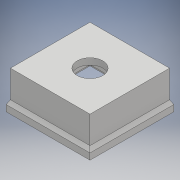
# Autodesk Inventor part: lupa_camera_mount
Saved by Autodesk Inventor 2018 (Build 220112000, 112)
## iProperties
Created: 2018-01-19
Part Number: lupa_camera_mount
Material: Generic
Document SubType Name: Modeling
Designer: matth
Density: 1 g/cm^3
Appearance: Default
Author: matth
Autodesk Inventor part; units mm, degrees
ref_plane "YZ Plane" through (0, 0, 0) normal (1, 0, 0) x (0, 1, 0)
ref_plane "XZ Plane" through (0, 0, 0) normal (0, 1, 0) x (-1, 0, 0)
ref_plane "XY Plane" through (0, 0, 0) normal (0, 0, 1) x (1, 0, 0)
sketch "Sketch1" plane through (0, 0, 0) normal (0, 0, 1) x (1, 0, 0)
  line L0 (-11.7234, 6.1825) -> (23.1766, 6.1825)
  line L1 (23.1766, 6.1825) -> (23.1766, -28.7175)
  line L2 (23.1766, -28.7175) -> (-11.7234, -28.7175)
  line L3 (-11.7234, -28.7175) -> (-11.7234, 6.1825)
  line L4 (-13.2234, 7.6825) -> (24.6766, 7.6825)
  line L5 (24.6766, 7.6825) -> (24.6766, -30.2175)
  line L6 (24.6766, -30.2175) -> (-13.2234, -30.2175)
  line L7 (-13.2234, -30.2175) -> (-13.2234, 7.6825)
  point P0 (0, 0)
  dimension "d0" = 34.9
  dimension "d1" = 34.9
  dimension "d2" = 37.9
  dimension "d3" = 37.9
  dimension "d4" = 1.5
  dimension "d5" = 1.5
  constraints: 16 end point, 4 parallel, 2 horizontal, 2 perpendicular
  measures "d0" distance of L1.end L2.end
  measures "d1" distance of L0.end L1.end
  measures "d2" distance of L5.end L6.end
  measures "d3" distance of L4.end L5.end
  measures "d4" distance between parallel lines of L4 L0
  measures "d5" distance between parallel lines of L7 L3
extrude "Extrusion1" add sketch "Sketch1" along normal blind 15
sketch "Sketch2" plane through (0, 0, 15) normal (0, 0, 1) x (1, 0, 0)
  line L0 (-13.2234, -30.2175) -> (-13.2234, 7.6825) projected
  line L1 (-13.2234, -30.2175) -> (24.6766, -30.2175) projected
  line L2 (-13.2234, 7.6825) -> (24.6766, 7.6825)
  line L3 (24.6766, 7.6825) -> (24.6766, -30.2175)
  line L4 (24.6766, -30.2175) -> (-13.2234, -30.2175)
  line L5 (-13.2234, -30.2175) -> (-13.2234, 7.6825)
  point P0 (0, 0)
  constraints: 8 end point, 2 parallel, 1 horizontal, 1 perpendicular
extrude "Extrusion2" add sketch "Sketch2" along normal blind 1
sketch "Sketch3" plane through (0, 0, 16) normal (0, 0, 1) x (1, 0, 0)
  circle A0 centre (5.7266, -11.2675) radius 6.1
  line L0 (-13.2234, 7.6825) -> (-13.2234, -30.2175) projected
  line L1 (-13.2234, -30.2175) -> (24.6766, -30.2175) projected
  point P0 (0, 0)
  dimension "d10" = 12.2
  dimension "d11" = 18.95
  dimension "d12" = 18.95
  dimension "d13" = 37.9
  constraints: 1 centre point
  measures "d10" diameter of A0
  measures "d11" distance from line of L0 A0.centre
  measures "d12" distance from line of L1 A0.centre
  measures "d13" distance of L0.start L0.end
extrude "Extrusion3" cut sketch "Sketch3" against normal blind 1
sketch "Sketch4" plane through (0, 0, 15) normal (0, 0, -1) x (-1, 0, 0)
  circle A0 centre (-5.7266, -11.2675) radius 6.1 projected
  circle A1 centre (-5.7266, -11.2675) radius 7.1
  point P0 (0, 0)
  dimension "d16" = 14.2
  constraints: 1 centre point, 1 coincident
  measures "d16" diameter of A1
extrude "Extrusion4" add sketch "Sketch4" along normal blind 2
sketch "Sketch5" plane through (0, 0, 0) normal (0, 0, -1) x (-1, 0, 0)
  line L0 (-24.6766, 7.6825) -> (-24.6766, -30.2175) projected
  line L1 (-24.6766, -30.2175) -> (13.2234, -30.2175) projected
  line L2 (13.2234, -30.2175) -> (13.2234, 7.6825) projected
  line L3 (13.2234, 7.6825) -> (-24.6766, 7.6825) projected
  line L4 (-25.6766, -31.2175) -> (14.2234, -31.2175)
  line L5 (14.2234, -31.2175) -> (14.2234, 8.6825)
  line L6 (14.2234, 8.6825) -> (-25.6766, 8.6825)
  line L7 (-25.6766, 8.6825) -> (-25.6766, -31.2175)
  point P0 (0, 0)
  dimension "d19" = 1
  dimension "d20" = 1
  dimension "d21" = 1
  dimension "d22" = 1
  constraints: 8 end point, 2 parallel, 1 horizontal, 1 perpendicular
  measures "d19" distance between parallel lines of L4 L1
  measures "d20" distance between parallel lines of L5 L2
  measures "d21" distance between parallel lines of L6 L3
  measures "d22" distance between parallel lines of L7 L0
extrude "Extrusion5" add sketch "Sketch5" along normal blind 2
sketch "Sketch6" plane through (0, 0, 0) normal (0, 0, 1) x (1, 0, 0)
  line L0 (-13.2234, 7.6825) -> (24.6766, 7.6825) projected
  line L1 (24.6766, 7.6825) -> (24.6766, -30.2175) projected
  line L2 (24.6766, -30.2175) -> (-13.2234, -30.2175) projected
  line L3 (-13.2234, -30.2175) -> (-13.2234, 7.6825) projected
  line L4 (25.6766, -31.2175) -> (-14.2234, -31.2175) projected
  line L5 (25.6766, 8.6825) -> (25.6766, -31.2175) projected
  line L6 (-14.2234, 8.6825) -> (25.6766, 8.6825) projected
  line L7 (-14.2234, -31.2175) -> (-14.2234, 8.6825) projected
  circle A0 centre (5.7266, -11.2675) radius 6.1 projected
  line L8 (24.6766, -30.2175) -> (24.6766, 7.6825) projected
  line L9 (24.6766, 7.6825) -> (-13.2234, 7.6825) projected
  line L10 (-13.2234, 7.6825) -> (-13.2234, -30.2175) projected
  line L11 (-13.2234, -30.2175) -> (24.6766, -30.2175) projected
  line L12 (24.6766, 7.6825) -> (-13.2234, 7.6825) projected
  point P0 (0, 0)
extrude "Extrusion6" add sketch "Sketch6" along normal blind 1 contours L4 L7 L6 L5
chamfer "Chamfer1" distance 2 distance2 1 1 edges at (-13.2234, -11.2675, 1) measured on face at (-13.2234, -11.2675, 1.5)
chamfer "Chamfer2" distance 2 distance2 1 2 edges at (-13.7233, -30.2175, 1) (5.7266, -30.2175, 1) measured on face at (-13.7233, -30.2175, 1.5) measured on face at (5.7266, -30.2175, 1.5)
chamfer "Chamfer3" distance 2 distance2 1 2 edges at (24.6766, -30.7175, 1) (24.6766, -11.2675, 1) measured on face at (24.6766, -30.7175, 1.5) measured on face at (24.6766, -11.2675, 1.5)
chamfer "Chamfer4" distance 2 distance2 1 3 edges at (25.1766, 7.6825, 1) (5.7266, 7.6825, 1) (-13.7233, 7.6825, 1) measured on face at (-13.7233, 7.6825, 1.5) measured on face at (5.7266, 7.6825, 1.5) measured on face at (25.1766, 7.6825, 1.5)
equation "\"d11\" = 0.5 * d13"
equation "\"d12\" = 0.5 * d13"
body "Solid1"
